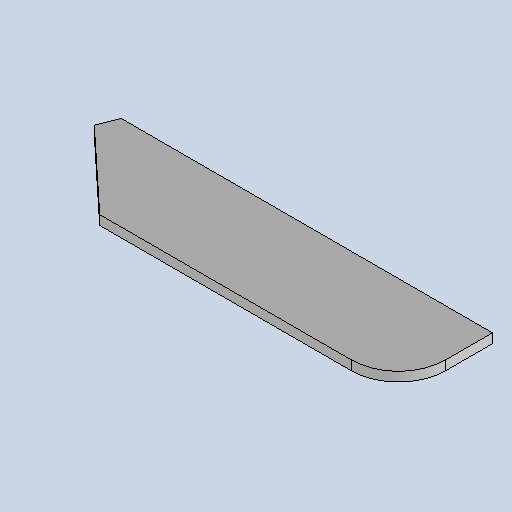
# Autodesk Inventor part: MSC 125 ROСKET PILLAR
Saved by Autodesk Inventor 2025 (Build 290162010, 162A)
## iProperties
Created: 2024-05-19
Part Number: MSC 125 ROСKET PILLAR
Material: Stainless Steel
Document SubType Name: Sheet Metal
Designer: admin
Stock Number: МОО 103 ракета нос
Mass: 9.29146 g
Surface Area: 30.5237 cm^2
Volume: 1.16143 cm^3
Density: 8 g/cm^3
Sheet Metal Rule: AISI304 2mm Die16
Sheet Metal Width: 20,000 mm
Sheet Metal Length: 80,612 mm
Sheet Metal Area: 1612,238 mm^2
Appearance: Default
Flat Pattern Width: 2 cm
Flat Pattern Length: 8.06119 cm
Flat Pattern Area: 16.1224 cm^2
Author: admin
Autodesk Inventor part; units mm, degrees
ref_plane "YZ Plane" through (0, 0, 0) normal (1, 0, 0) x (0, 1, 0)
ref_plane "XZ Plane" through (0, 0, 0) normal (0, 1, 0) x (-1, 0, 0)
ref_plane "XY Plane" through (0, 0, 0) normal (0, 0, 1) x (1, 0, 0)
sketch "Sketch2" plane through (0, 0, 0) normal (0, 0, 1) x (1, 0, 0)
  line L0 (0, 0) -> (0, 20)
  line L1 (0, 20) -> (-85, 20)
  line L2 (-85, 20) -> (-85, 0)
  line L3 (-85, 0) -> (0, 0)
  line L4 (-85, 20) -> (-63.5526, 0)
  dimension "d10" = 20
  dimension "d30" = 85
  dimension "d31" = 43
  measures "d10" distance of L0.start L0.end
  measures "d30" distance of L0.end L1.end
  measures "d31" angle of L1 L4
extrude "Plate1" add sketch "Sketch2" along normal blind 2 contours L3 L4 L1 L0
fillet "Corner Round2" radius 10 1 edges at (0, 0, 1)
chamfer "Corner Chamfer1" distance 6 angle 45 1 edges at (-85, 20, 1)
equation "\"d7\" = Thickness"
equation "\"BendReliefWidth\" = Thickness"
equation "\"BendReliefDepth\" = 0.5 * Thickness"
equation "\"CornerReliefSize\" = 4 * Thickness"
equation "\"MinimumRemnant\" = 2 * Thickness"
equation "\"TransitionRadius\" = BendRadius"
equation "\"JacobiRadiusSize\" = BendRadius"
equation "\"GapSize\" = Thickness"
equation "\"Thickness\" = 2"
equation "\"BendRadius\" = 2.75"
body "Solid2"
